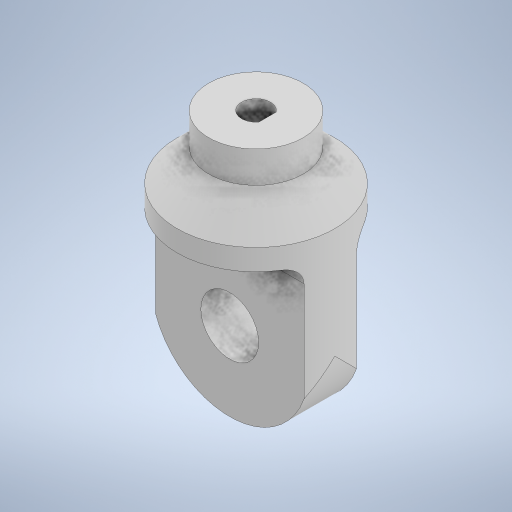
# Autodesk Inventor part: 회전대
Saved by Autodesk Inventor 2023 (Build 270158000, 158)
## iProperties
Created: 2022-11-11
Part Number: 회전대
Material: 일반
Document SubType Name: Modeling
Designer: hyunsu
Density: 1 g/cm^3
Appearance: 기본값
Author: hyunsu
Autodesk Inventor part; units mm, degrees
ref_plane "YZ Plane" through (0, 0, 0) normal (1, 0, 0) x (0, 1, 0)
ref_plane "XZ Plane" through (0, 0, 0) normal (0, 1, 0) x (-1, 0, 0)
ref_plane "XY Plane" through (0, 0, 0) normal (0, 0, 1) x (1, 0, 0)
sketch "스케치1" plane through (0, 0, 0) normal (0, 1, 0) x (-1, 0, 0)
  circle A0 centre (0, 0) radius 15
  dimension "d0" = 30
  constraints: 1 centre point, 1 coincident
  measures "d0" diameter of A0
extrude "돌출1" add sketch "스케치1" against normal blind 10
sketch "스케치2" plane through (0, -10, 0) normal (0, -1, 0) x (1, 0, 0)
  circle A0 centre (0, 0) radius 15 projected
  circle A1 centre (0, 0) radius 15 projected
  line L0 (-14.1421, 5) -> (14.1421, 5)
  line L1 (0, 0) -> (4.8665, 0)
  line L2 (-14.1421, -5) -> (14.1421, -5)
  dimension "d3" = 10
  constraints: 6 end point, 2 horizontal, 2 point on circle, 2 symmetric about line
  measures "d3" distance between parallel lines of L0 L2
extrude "돌출2" add sketch "스케치2" along normal blind 32 contours A0 L2 L0
sketch "스케치3" plane through (-14.1421, -10, 5) normal (0, 0, 1) x (1, 0, 0)
  circle A0 centre (14.1421, -17) radius 15
  line L0 (28.2843, -32) -> (0, -32) projected
  line L1 (-0.8579, -2) -> (29.1421, -2)
  line L2 (29.1421, -2) -> (29.1421, -32)
  line L3 (29.1421, -32) -> (-0.8579, -32)
  line L4 (-0.8579, -32) -> (-0.8579, -2)
  line L5 (-0.8579, -2) -> (29.1421, -32) construction
  line L6 (29.1421, -2) -> (-0.8579, -32) construction
  line L7 (28.2843, -32) -> (29.1421, -32) projected
  point P0 (14.1421, 10)
  point P1 (14.1421, -32)
  point P2 (-0.8579, -17)
  point P3 (14.1421, -32)
  point P4 (29.1421, -17)
  dimension "d6" = 30
  constraints: 12 end point, 3 midpoint, 2 parallel, 2 tangent, 1 centre point, 1 horizontal, 1 perpendicular, 1 point on line, 1 vertical alignment
  measures "d6" diameter of A0
extrude "돌출3" cut sketch "스케치3" against normal blind 32 contours L2 L3 L0 A0 | L0 L3 L4 A0
chamfer "모따기1" distance 6 angle 45 1 edges at (15, 0, 0) measured on face at (14.5, 0, 0)
fillet "모깎기1" radius 3 2 edges at (0, -10, -5) (0, -10, 5)
sketch "스케치4" plane through (0, 0, 0) normal (1, 0, 0) x (0, 1, 0)
  line L0 (-41.9354, -5) -> (-11.9354, -5)
  line L1 (-13, -5) -> (-32, -5) projected
  line L2 (-42, -5) -> (-32, -5) projected
  circle A0 centre (-37.9354, -5) radius 1.15
  point P0 (0, 0)
  point P1 (-26.9354, -5)
  point P2 (-36.7854, -5)
  point P3 (-39.0854, -5)
  dimension "d15" = 30
  dimension "d16" = 2.3
  dimension "d17" = 11
  constraints: 2 end point, 1 centre point, 1 collinear, 1 midpoint, 1 point on line
  measures "d15" distance of L0.start L0.end
  measures "d16" diameter of A0
  measures "d17" distance of point (-26.935, -5) A0.centre
revolve "회전1" cut sketch "스케치4" angle 360 about axis through (0, -41.9354, -5) along (0, 1, 0) picked at (-37.8892, -4.6195) contours A0 L0
sketch "스케치5" plane through (0, -27, -5) normal (0, 0, -1) x (-1, 0, 0)
  circle A0 centre (0, 0) radius 5.5
  arc A1 (-14.1421, -5) -> (14.1421, -5) centre (0, 0) ccw projected
  point P0 (0, 27)
  dimension "d19" = 11
  constraints: 1 centre point, 1 coincident
  measures "d19" diameter of A0
extrude "돌출4" cut sketch "스케치5" against normal blind 32
pattern_circular "원형 패턴1" count 20 over 360 about axis through (0, -27, -5) along (0, 0, 1) of "회전1"
sketch "스케치6" plane through (0, 0, 0) normal (0, 1, 0) x (1, 0, 0)
  circle A0 centre (0, 0) radius 9 projected
extrude "돌출5" add sketch "스케치6" along normal blind 6
sketch "스케치7" plane through (0, 6, 0) normal (0, 1, 0) x (1, 0, 0)
  circle A0 centre (0, 0) radius 2.75
  line L0 (2.2, 1.65) -> (2.2, -1.65)
  dimension "d27" = 5.5
  dimension "d28" = 2.2
  constraints: 2 end point, 2 point on circle, 1 centre point, 1 coincident, 1 vertical
  measures "d27" diameter of A0
  measures "d28" distance from line of point (0, 0) L0
extrude "돌출6" cut sketch "스케치7" against normal blind 20 contours L0 A0 picked at (-0.2276, -0.7952)
